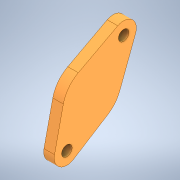
# Autodesk Inventor part: frame_center
Saved by Autodesk Inventor 2021 (Build 250183000, 183)
## iProperties
Created: 2022-05-14
Part Number: frame_center
Material: Generic
Document SubType Name: Modeling
Designer: ermoz
Density: 1 g/cm^3
Appearance: Default
Author: ermoz
Autodesk Inventor part; units mm, degrees
ref_plane "YZ Plane" through (0, 0, 0) normal (1, 0, 0) x (0, 1, 0)
ref_plane "XZ Plane" through (0, 0, 0) normal (0, 1, 0) x (-1, 0, 0)
ref_plane "XY Plane" through (0, 0, 0) normal (0, 0, 1) x (1, 0, 0)
sketch "Sketch3" plane through (0, 0, 0) normal (1, 0, 0) x (0, 1, 0)
  circle A0 centre (0, 0) radius 14
  line L0 (-23, -102.8316) -> (23, -102.8316)
  line L1 (23, -102.8316) -> (23, 102.8316)
  line L2 (23, 102.8316) -> (-23, 102.8316)
  line L3 (-23, 102.8316) -> (-23, -102.8316)
  line L4 (-23, -102.8316) -> (23, 102.8316) construction
  line L5 (23, -102.8316) -> (-23, 102.8316) construction
  circle A1 centre (17, -15) radius 2.5
  circle A2 centre (-17, 12) radius 2.5
  circle A3 centre (17, -15) radius 6
  circle A4 centre (-17, 12) radius 6
  line L6 (-22.0787, 8.8052) -> (-11.8503, -7.4546)
  line L7 (-4.9626, -13.0909) -> (14.8732, -20.6104)
  line L8 (12.3712, 6.554) -> (22.3019, -12.1912)
  line L9 (3.0558, 13.6624) -> (-15.6904, 17.8553)
  dimension "d11" = 28
  dimension "d12" = 46
  dimension "d13" = 5
  dimension "d14" = 6
  dimension "d15" = 6
  dimension "d16" = 12
  dimension "d17" = 15
  constraints: 20 end point, 10 tangent, 8 point on circle, 5 centre point, 3 coincident, 2 midpoint, 2 parallel, 2 perpendicular, 1 equal radius, 1 horizontal
  measures "d11" diameter of A0
  measures "d12" distance of L1.end L2.end
  measures "d13" diameter of A1
  measures "d14" distance from line of L3 A2.centre
  measures "d15" distance from line of L1 A1.centre
  measures "d16" vertical distance of A2.centre point (0, 0)
  measures "d17" vertical distance of A1.centre point (0, 0)
extrude "Extrusion3" add sketch "Sketch3" along normal blind 5 contours A0 | A0 L8 A3 L7 | A0 L6 A4 L9 | A3 | A4
body "Solid2"
